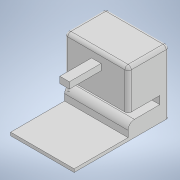
# Autodesk Inventor part: Royce 610 Base
Saved by Autodesk Inventor 2022 (Build 260153000, 153)
## iProperties
Created: 2022-02-10
Part Number: Royce 610 Base
Material: Generic
Document SubType Name: Modeling
Designer: Caleb
Density: 1 g/cm^3
Appearance: Default
Author: Caleb
Autodesk Inventor part; units mm, degrees
ref_plane "YZ Plane" through (0, 0, 0) normal (1, 0, 0) x (0, 1, 0)
ref_plane "XZ Plane" through (0, 0, 0) normal (0, 1, 0) x (-1, 0, 0)
ref_plane "XY Plane" through (0, 0, 0) normal (0, 0, 1) x (1, 0, 0)
sketch "Sketch1" plane through (0, 0, 0) normal (0, 1, 0) x (-1, 0, 0)
  line L0 (-127, -190.5) -> (127, -190.5)
  line L1 (127, -190.5) -> (127, 190.5)
  line L2 (127, 190.5) -> (-127, 190.5)
  line L3 (-127, 190.5) -> (-127, -190.5)
  line L4 (-127, -190.5) -> (127, 190.5) construction
  line L5 (127, -190.5) -> (-127, 190.5) construction
  point P0 (0, 0)
  dimension "d0" = 254
  dimension "d1" = 381
  constraints: 12 end point, 2 midpoint, 2 parallel, 1 horizontal, 1 perpendicular
  measures "d0" distance of L1.end L2.end
  measures "d1" distance of L0.end L1.end
extrude "Extrusion1" add sketch "Sketch1" along normal blind 254
sketch "Sketch2" plane through (127, 0, 190.5) normal (1, 0, 0) x (0, 0, -1)
  line L0 (0, 0) -> (0, 254) projected
  line L1 (0, 12.7) -> (215.9, 12.7)
  line L2 (0, 12.7) -> (215.9, 12.7) construction
  line L3 (215.9, 12.7) -> (215.9, 38.1)
  line L4 (0, 0) -> (381, 0) projected
  arc A0 (241.3, 63.5) -> (215.9, 38.1) centre (241.3, 38.1) ccw
  line L5 (241.3, 63.5) -> (342.9, 63.5)
  line L6 (342.9, 63.5) -> (342.9, 95.25)
  line L7 (342.9, 95.25) -> (215.9, 95.25)
  line L8 (215.9, 95.25) -> (215.9, 190.5)
  line L9 (215.9, 190.5) -> (88.9, 190.5)
  line L10 (88.9, 190.5) -> (88.9, 215.9)
  line L11 (88.9, 215.9) -> (215.9, 215.9)
  line L12 (215.9, 215.9) -> (215.9, 254)
  line L13 (381, 254) -> (0, 254) projected
  point P0 (190.5, 0)
  dimension "d4" = 215.9
  dimension "d6" = 25.4
  dimension "d7" = 12.7
  dimension "d8" = 25.4
  dimension "d9" = 101.6
  dimension "d10" = 31.75
  dimension "d11" = 25.4
  dimension "d12" = 177.8
  dimension "d13" = 25.4
  dimension "d14" = 127
  constraints: 22 end point, 7 perpendicular, 4 point on line, 2 horizontal, 2 point on circle, 1 centre point, 1 collinear, 1 tangent, 1 vertical, 1 vertical alignment
  measures "d4" distance of L1.start L1.end
  measures "d6" distance of L1.end L3.end
  measures "d7" distance between parallel lines of L4 L1
  measures "d8" radius of A0
  measures "d9" distance of L5.start L5.end
  measures "d10" distance of L5.end L6.end
  measures "d11" horizontal distance of L3.end L5.start
  measures "d12" distance between parallel lines of L1 L9
  measures "d13" distance of L9.end L10.end
  measures "d14" distance of L8.end L9.end
extrude "Extrusion2" cut sketch "Sketch2" against normal through all
sketch "Sketch3" plane through (127, 215.9, 101.6) normal (0, 1, 0) x (1, 0, 0)
  line L0 (-254, 127) -> (0, 127) projected
  line L1 (-254, -88.9) -> (-146.05, -88.9)
  line L2 (-146.05, -88.9) -> (-146.05, 127)
  line L3 (-146.05, 127) -> (-254, 127)
  line L4 (-254, 127) -> (-254, -88.9)
  line L5 (0, -88.9) -> (0, 292.1) projected
  line L6 (0, -88.9) -> (-107.95, -88.9)
  line L7 (-107.95, -88.9) -> (-107.95, 127)
  line L8 (-107.95, 127) -> (0, 127)
  line L9 (0, 127) -> (0, -88.9)
  point P0 (-127, 101.6)
  point P1 (-254, 127)
  dimension "d17" = 38.1
  constraints: 16 end point, 4 parallel, 2 horizontal, 2 perpendicular, 2 point on line, 1 collinear
  measures "d17" distance between parallel lines of L2 L7
extrude "Extrusion3" cut sketch "Sketch3" against normal blind 25.4
sketch "Sketch4" plane through (-19.05, 190.5, -25.4) normal (0, -1, 0) x (1, 0, 0)
  circle A0 centre (19.05, 111.125) radius 3.175
  line L0 (38.1, 0) -> (0, 0) projected
  line L1 (38.1, 0) -> (38.1, 127) projected
  point P0 (19.05, 25.4)
  dimension "d20" = 6.35
  dimension "d21" = 111.125
  dimension "d22" = 19.05
  constraints: 1 centre point
  measures "d20" diameter of A0
  measures "d21" distance from line of L0 A0.centre
  measures "d22" distance from line of L1 A0.centre
extrude "Extrusion4" add sketch "Sketch4" along normal blind 25.4
fillet "Fillet1" radius 12.7 8 edges at (0, 254, -25.4) (127, 174.625, -25.4) (127, 254, -107.95) (-127, 174.625, -25.4) (-127, 254, -107.95) (127, 127, -190.5) (0, 254, -190.5) (-127, 127, -190.5)
body "Solid1"
